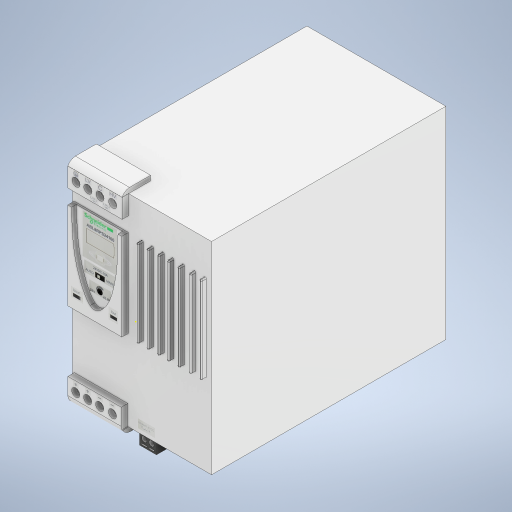
# Autodesk Inventor part: napojna_jedinica_ABL8RPS24100
Saved by Autodesk Inventor 2023 (Build 270158000, 158)
## iProperties
Created: 2022-07-15
Part Number: napojna_jedinica_ABL8RPS24100
Material: Generic
Document SubType Name: Sheet Metal
Designer: User
Density: 1 g/cm^3
Sheet Metal Rule: Default
Appearance: Default
Author: User
Autodesk Inventor part; units mm, degrees
ref_plane "YZ Plane" through (0, 0, 0) normal (1, 0, 0) x (0, 1, 0)
ref_plane "XZ Plane" through (0, 0, 0) normal (0, 1, 0) x (-1, 0, 0)
ref_plane "XY Plane" through (0, 0, 0) normal (0, 0, 1) x (1, 0, 0)
sketch "Sketch1" plane through (0, 0, 0) normal (0, 0, 1) x (1, 0, 0)
  line L0 (43, -62.5) -> (-43, -62.5)
  line L1 (-43, -62.5) -> (-43, 62.5)
  line L2 (-43, 62.5) -> (43, 62.5)
  line L3 (43, 62.5) -> (43, -62.5)
  line L4 (43, -62.5) -> (-43, 62.5) construction
  line L5 (-43, -62.5) -> (43, 62.5) construction
  point P0 (0, 0)
  dimension "d0" = 125
  dimension "d1" = 86
  constraints: 12 end point, 2 midpoint, 2 parallel, 1 horizontal, 1 perpendicular
  measures "d0" distance of L0.end L1.end
  measures "d1" distance of L1.end L2.end
extrude "Extrusion1" add sketch "Sketch1" against normal blind 145
sketch "Sketch2" plane through (0, 0, 0) normal (0, 0, 1) x (1, 0, 0)
  line L0 (-8.4534, -12.4164) -> (-42.0011, -12.4164)
  line L1 (-42.0011, -12.4164) -> (-42.0011, 41.6134)
  line L2 (-42.0011, 41.6134) -> (-8.4534, 41.6134)
  line L3 (-8.4534, 41.6134) -> (-8.4534, -12.4164)
  line L4 (-8.4534, -12.4164) -> (-42.0011, 41.6134) construction
  line L5 (-42.0011, -12.4164) -> (-8.4534, 41.6134) construction
  line L6 (-8.3237, 50.7106) -> (-41.8747, 50.7106)
  line L7 (-41.8747, 50.7106) -> (-41.8747, 62.4919)
  line L8 (-41.8747, 62.4919) -> (-8.3237, 62.4919)
  line L9 (-8.3237, 62.4919) -> (-8.3237, 50.7106)
  line L10 (-8.3237, 50.7106) -> (-41.8747, 62.4919) construction
  line L11 (-41.8747, 50.7106) -> (-8.3237, 62.4919) construction
  line L12 (-41.8747, -50.1984) -> (-8.8359, -50.1984)
  line L13 (-8.8359, -50.1984) -> (-8.8359, -62.748)
  line L14 (-8.8359, -62.748) -> (-41.8747, -62.748)
  line L15 (-41.8747, -62.748) -> (-41.8747, -50.1984)
  line L16 (-41.8747, -50.1984) -> (-8.8359, -62.748) construction
  line L17 (-8.8359, -50.1984) -> (-41.8747, -62.748) construction
  line L18 (0.7683, -12.3428) -> (-0.7683, -12.3428)
  line L19 (-0.7683, -12.3428) -> (-0.7683, 41.6871)
  line L20 (-0.7683, 41.6871) -> (0.7683, 41.6871)
  line L21 (0.7683, 41.6871) -> (0.7683, -12.3428)
  line L22 (0.7683, -12.3428) -> (-0.7683, 41.6871) construction
  line L23 (-0.7683, -12.3428) -> (0.7683, 41.6871) construction
  line L24 (26.2391, -12.3428) -> (24.7024, -12.3428)
  line L25 (24.7024, -12.3428) -> (24.7024, 41.6871)
  line L26 (24.7024, 41.6871) -> (26.2391, 41.6871)
  line L27 (26.2391, 41.6871) -> (26.2391, -12.3428)
  line L28 (26.2391, -12.3428) -> (24.7024, 41.6871) construction
  line L29 (24.7024, -12.3428) -> (26.2391, 41.6871) construction
  line L30 (19.7125, -12.3729) -> (18.1758, -12.3729)
  line L31 (18.1758, -12.3729) -> (18.1758, 41.7648)
  line L32 (18.1758, 41.7648) -> (19.7125, 41.7648)
  line L33 (19.7125, 41.7648) -> (19.7125, -12.3729)
  line L34 (19.7125, -12.3729) -> (18.1758, 41.7648) construction
  line L35 (18.1758, -12.3729) -> (19.7125, 41.7648) construction
  line L36 (33.3265, -12.2364) -> (31.7898, -12.2364)
  line L37 (31.7898, -12.2364) -> (31.7898, 41.6856)
  line L38 (31.7898, 41.6856) -> (33.3265, 41.6856)
  line L39 (33.3265, 41.6856) -> (33.3265, -12.2364)
  line L40 (33.3265, -12.2364) -> (31.7898, 41.6856) construction
  line L41 (31.7898, -12.2364) -> (33.3265, 41.6856) construction
  line L42 (5.5817, 41.7558) -> (7.1183, 41.7558)
  line L43 (5.5817, -12.3819) -> (5.5817, 41.7558)
  line L44 (7.1183, 41.7558) -> (7.1183, -12.3819)
  line L45 (5.5817, -12.3819) -> (7.1183, 41.7558) construction
  line L46 (7.1183, -12.3819) -> (5.5817, 41.7558) construction
  line L47 (7.1183, -12.3819) -> (5.5817, -12.3819)
  line L48 (38.2302, 41.6103) -> (39.7669, 41.6103)
  line L49 (38.2302, -12.3118) -> (38.2302, 41.6103)
  line L50 (39.7669, 41.6103) -> (39.7669, -12.3118)
  line L51 (38.2302, -12.3118) -> (39.7669, 41.6103) construction
  line L52 (39.7669, -12.3118) -> (38.2302, 41.6103) construction
  line L53 (39.7669, -12.3118) -> (38.2302, -12.3118)
  line L54 (12.1537, 41.8636) -> (13.6904, 41.8636)
  line L55 (12.1537, -12.2741) -> (12.1537, 41.8636)
  line L56 (13.6904, 41.8636) -> (13.6904, -12.2741)
  line L57 (12.1537, -12.2741) -> (13.6904, 41.8636) construction
  line L58 (13.6904, -12.2741) -> (12.1537, 41.8636) construction
  line L59 (13.6904, -12.2741) -> (12.1537, -12.2741)
  point P0 (0, 0)
  point P1 (-25.2272, 14.5985)
  point P2 (-25.0992, 56.6012)
  point P3 (-25.3553, -56.4732)
  point P4 (0, 14.6721)
  point P5 (1.5875, 1.5875)
  point P6 (25.4708, 14.6721)
  point P7 (3.175, 3.175)
  point P8 (18.9442, 14.696)
  point P9 (4.7625, 4.7625)
  point P10 (32.5581, 14.7246)
  point P11 (3.175, 3.175)
  point P12 (6.35, 14.6869)
  point P13 (4.7625, 4.7625)
  point P14 (38.9985, 14.6493)
  point P15 (6.35, 6.35)
  point P16 (12.9221, 14.7948)
  constraints: 120 end point, 20 midpoint, 20 parallel, 10 horizontal, 10 perpendicular
extrude "Extrusion2" add sketch "Sketch2" along normal blind 4 contours L0 L1 L2 L3
extrude "Extrusion3" add sketch "Sketch2" along normal blind 4 contours L6 L7 L8 L9 | L12 L13 L14 L15
extrude "Extrusion4" add sketch "Sketch2" along normal blind 3 contours L18 L19 L20 L21 | L24 L25 L26 L27 | L30 L31 L32 L33 | L36 L37 L38 L39 | L42 L44 L47 L43 | L48 L50 L53 L49 | L54 L56 L59 L55
fillet "Fillet1" radius 0.7 2 edges at (0.7683, 14.6721, 3) (-0.7683, 14.6721, 3)
fillet "Fillet2" radius 0.7 12 edges at (5.5817, 14.6869, 3) (7.1183, 14.6869, 3) (12.1537, 14.7948, 3) (13.6904, 14.7948, 3) (18.1758, 14.696, 3) (19.7125, 14.696, 3) (24.7024, 14.6721, 3) (26.2391, 14.6721, 3) (31.7898, 14.7246, 3) (33.3265, 14.7246, 3) (38.2302, 14.6493, 3) (39.7669, 14.6493, 3)
fillet "Fillet3" radius 0.7 35 edges at (38.9985, 41.6103, 3) (38.4352, 41.6103, 2.795) (38.2302, 41.6103, 1.15) (39.7669, 41.6103, 1.15) (39.5618, 41.6103, 2.795) (32.5581, 41.6856, 3) (31.9948, 41.6856, 2.795) (31.7898, 41.6856, 1.15) (33.3265, 41.6856, 1.15) (33.1215, 41.6856, 2.795) (25.4708, 41.6871, 3) (24.9075, 41.6871, 2.795) (24.7024, 41.6871, 1.15) (26.2391, 41.6871, 1.15) (26.0341, 41.6871, 2.795) (18.9442, 41.7648, 3) (18.3809, 41.7648, 2.795) (18.1758, 41.7648, 1.15) (19.7125, 41.7648, 1.15) (19.5075, 41.7648, 2.795) (12.9221, 41.8636, 3) (12.3588, 41.8636, 2.795) (12.1537, 41.8636, 1.15) (13.6904, 41.8636, 1.15) (13.4854, 41.8636, 2.795) (6.35, 41.7558, 3) (5.7867, 41.7558, 2.795) (5.5817, 41.7558, 1.15) (7.1183, 41.7558, 1.15) (6.9133, 41.7558, 2.795) (0, 41.6871, 3) (-0.5633, 41.6871, 2.795) (-0.7683, 41.6871, 1.15) (0.7683, 41.6871, 1.15) (0.5633, 41.6871, 2.795)
fillet "Fillet4" radius 0.7 35 edges at (0.7683, -12.3428, 1.15) (0, -12.3428, 3) (-0.5633, -12.3428, 2.795) (-0.7683, -12.3428, 1.15) (0.5633, -12.3428, 2.795) (7.1183, -12.3819, 1.15) (6.35, -12.3819, 3) (5.7867, -12.3819, 2.795) (5.5817, -12.3819, 1.15) (6.9133, -12.3819, 2.795) (13.6904, -12.2741, 1.15) (12.9221, -12.2741, 3) (12.3588, -12.2741, 2.795) (12.1537, -12.2741, 1.15) (13.4854, -12.2741, 2.795) (19.7125, -12.3729, 1.15) (18.9442, -12.3729, 3) (18.3809, -12.3729, 2.795) (18.1758, -12.3729, 1.15) (19.5075, -12.3729, 2.795) (24.9075, -12.3428, 2.795) (25.4708, -12.3428, 3) (26.0341, -12.3428, 2.795) (26.2391, -12.3428, 1.15) (24.7024, -12.3428, 1.15) (33.3265, -12.2364, 1.15) (32.5581, -12.2364, 3) (31.9948, -12.2364, 2.795) (31.7898, -12.2364, 1.15) (33.1215, -12.2364, 2.795) (39.7669, -12.3118, 1.15) (38.9985, -12.3118, 3) (38.4352, -12.3118, 2.795) (38.2302, -12.3118, 1.15) (39.5618, -12.3118, 2.795)
sketch "Sketch3" plane through (-43, 62.5, 0) normal (0, 1, 0) x (1, 0, 0)
  line L0 (34.6244, -3.9581) -> (1.0619, -3.9581)
  line L1 (1.0619, -3.9581) -> (1.0619, 13.6548)
  line L2 (1.0619, 13.6548) -> (34.6244, 13.6548)
  line L3 (34.6244, 13.6548) -> (34.6244, -3.9581)
  line L4 (34.6244, -3.9581) -> (1.0619, 13.6548) construction
  line L5 (1.0619, -3.9581) -> (34.6244, 13.6548) construction
  point P0 (43, 0)
  point P1 (17.8432, 4.8484)
  constraints: 12 end point, 2 midpoint, 2 parallel, 1 horizontal, 1 perpendicular
extrude "Extrusion5" add sketch "Sketch3" along normal blind 3
fillet "Fillet5" radius 5 1 edges at (-25.1568, 65.5, 3.9581)
sketch "Sketch4" plane through (-43, -62.5, -145) normal (0, -1, 0) x (1, 0, 0)
  line L0 (34.5466, 149) -> (0.9989, 149) projected
  line L1 (34.6874, 128.9171) -> (0.9989, 128.9171)
  line L2 (0.9989, 128.9171) -> (0.9989, 149)
  line L3 (0.9989, 149) -> (34.6874, 149)
  line L4 (34.6874, 149) -> (34.6874, 128.9171)
  line L5 (34.6874, 128.9171) -> (0.9989, 149) construction
  line L6 (0.9989, 128.9171) -> (34.6874, 149) construction
  point P0 (43, 145)
  point P1 (17.8432, 138.9585)
  constraints: 12 end point, 2 midpoint, 2 parallel, 1 horizontal, 1 perpendicular
extrude "Extrusion6" add sketch "Sketch4" along normal blind 3
fillet "Fillet6" radius 5 1 edges at (-25.1568, -65.5, 4)
sketch "Sketch5" plane through (0, 0, 4) normal (0, 0, 1) x (1, 0, 0)
  point P0 (0, 0)
sketch "Sketch6" plane through (0, 0, 4) normal (0, 0, 1) x (1, 0, 0)
  line L0 (-42.0134, 40.8092) -> (-7.5398, 40.8092) construction
  line L1 (-7.5398, 40.8092) -> (-7.5398, -8.8157) construction
  line L2 (-7.5398, -8.8157) -> (-42.0134, -8.8157) construction
  line L3 (-42.0134, -8.8157) -> (-42.0134, 40.8092) construction
  line L4 (-42.0011, 41.6134) -> (-8.4534, 41.6134) projected
  spline S0 degree 4 poles (-39.6427, 41.6134) (-39.5386, 39.0441) (-39.1974, 21.8727) (-37.9398, 12.4752) (-31.2758, -3.0074) (-28.1197, -5.3577) knots 0 0 0 0 0 0.490778 1 1 1 1 1
  spline S1 degree 4 poles (-10.883, 41.6134) (-10.9429, 39.1847) (-10.7419, 26.6675) (-12.0599, 17.1608) (-16.3516, -0.707) (-22.8529, -6.5254) (-25.813, -7.2256) (-28.1197, -5.3577) knots 0 0 0 0 0 0.398035 0.568703 0.718295 1 1 1 1 1
  line L5 (-39.6427, 41.6134) -> (-10.883, 41.6134)
  point P0 (0, 0)
  point P1 (-39.4451, 35.6169)
  point P2 (-38.6549, 23.4672)
  point P3 (-36.5806, 12.1076)
  point P4 (-32.4319, 0.8469)
  point P5 (-10.9341, 35.6169)
  point P6 (-11.5549, 23.4671)
  point P7 (-13.4008, 12.1076)
  point P8 (-17.2522, 0.8469)
  point P9 (-22.0273, -4.981)
  point P10 (-25.2273, -6.4217)
  constraints: 2 end point, 2 point on line, 1 collinear, 16 other
extrude "Extrusion7" cut sketch "Sketch6" against normal blind 3
sketch "Sketch7" plane through (0, 0, 1) normal (0, 0, 1) x (1, 0, 0)
  line L0 (-35.8459, 40.4822) -> (-14.5747, 40.4822) construction
  line L1 (-14.5747, 40.4822) -> (-14.5747, 15.9143) construction
  line L2 (-14.5747, 15.9143) -> (-35.8459, 15.9143) construction
  line L3 (-35.8459, 15.9143) -> (-35.8459, 40.4822) construction
  line L4 (-34.7955, 14.6387) -> (-15.0999, 14.6387) construction
  line L5 (-15.0999, 14.6387) -> (-15.0999, 7.9537) construction
  line L6 (-15.0999, 7.9537) -> (-34.7955, 7.9537) construction
  line L7 (-34.7955, 7.9537) -> (-34.7955, 14.6387) construction
  line L8 (-31.6442, 5.4452) -> (-18.2512, 5.4452) construction
  line L9 (-18.2512, 5.4452) -> (-18.2512, -0.4276) construction
  line L10 (-18.2512, -0.4276) -> (-31.6442, -0.4276) construction
  line L11 (-31.6442, -0.4276) -> (-31.6442, 5.4452) construction
  point P0 (0, 0)
  constraints: 6 other
decal "Decal1"
decal "Decal2"
decal "Decal3"
sketch "Sketch8" plane through (0, 0, 4) normal (0, 0, 1) x (1, 0, 0)
  line L0 (-16.7418, -0.0611) -> (-10.8655, -0.0611) construction
  line L1 (-10.8655, -0.0611) -> (-10.8655, -6.9406) construction
  line L2 (-10.8655, -6.9406) -> (-16.7418, -6.9406) construction
  line L3 (-16.7418, -6.9406) -> (-16.7418, -0.0611) construction
  line L4 (-39.8987, -0.6259) -> (-32.597, -0.6259) construction
  line L5 (-32.597, -0.6259) -> (-32.597, -6.5585) construction
  line L6 (-32.597, -6.5585) -> (-39.8987, -6.5585) construction
  line L7 (-39.8987, -6.5585) -> (-39.8987, -0.6259) construction
  point P0 (0, 0)
  constraints: 4 other
decal "Decal4"
decal "Decal5"
sketch "Sketch9" plane through (0, 0, 4) normal (0, 0, 1) x (1, 0, 0)
  circle A0 centre (-36.8873, 56.3383) radius 2.54
  circle A1 centre (-29.4981, 56.3383) radius 2.54
  circle A2 centre (-22.0468, 56.3383) radius 2.54
  circle A3 centre (-14.1608, 56.3383) radius 2.54
  point P0 (0, 0)
  dimension "d117" = 5.08
  dimension "d118" = 5.08
  dimension "d119" = 5.08
  dimension "d120" = 5.08
  constraints: 4 centre point
  measures "d117" diameter of A0
  measures "d118" diameter of A1
  measures "d119" diameter of A2
  measures "d120" diameter of A3
sketch "Sketch10" plane through (0, 0, 4) normal (0, 0, 1) x (1, 0, 0)
  circle A0 centre (-37.0437, -56.4262) radius 2.54
  circle A1 centre (-29.6545, -56.4262) radius 2.54
  circle A2 centre (-22.2032, -56.4262) radius 2.54
  circle A3 centre (-14.3172, -56.4262) radius 2.54
  point P0 (0, 0)
  dimension "d121" = 5.08
  dimension "d122" = 5.08
  dimension "d123" = 5.08
  dimension "d124" = 5.08
  constraints: 4 centre point
  measures "d121" diameter of A0
  measures "d122" diameter of A1
  measures "d123" diameter of A2
  measures "d124" diameter of A3
extrude "Extrusion8" cut sketch "Sketch9" against normal blind 3
extrude "Extrusion9" cut sketch "Sketch10" against normal blind 3
sketch "Sketch11" plane through (0, 0, 4) normal (0, 0, 1) x (1, 0, 0)
  line L0 (-31.3238, -50.4843) -> (-27.885, -50.4843) construction
  line L1 (-27.885, -50.4843) -> (-27.885, -53.5793) construction
  line L2 (-27.885, -53.5793) -> (-31.3238, -53.5793) construction
  line L3 (-31.3238, -53.5793) -> (-31.3238, -50.4843) construction
  line L4 (-38.6549, -50.5658) -> (-35.3066, -50.5658) construction
  line L5 (-35.3066, -50.5658) -> (-35.3066, -53.5793) construction
  line L6 (-35.3066, -53.5793) -> (-38.6549, -53.5793) construction
  line L7 (-38.6549, -53.5793) -> (-38.6549, -50.5658) construction
  line L8 (-16.3901, -50.587) -> (-12.4983, -50.587) construction
  line L9 (-12.4983, -50.587) -> (-12.4983, -53.2729) construction
  line L10 (-12.4983, -53.2729) -> (-16.3901, -53.2729) construction
  line L11 (-16.3901, -53.2729) -> (-16.3901, -50.587) construction
  line L12 (-24.1737, -50.656) -> (-20.1914, -50.656) construction
  line L13 (-20.1914, -50.656) -> (-20.1914, -53.4044) construction
  line L14 (-20.1914, -53.4044) -> (-24.1737, -53.4044) construction
  line L15 (-24.1737, -53.4044) -> (-24.1737, -50.656) construction
  point P0 (0, 0)
  constraints: 8 other
decal "Decal6"
decal "Decal7"
decal "Decal8"
decal "Decal9"
sketch "Sketch12" plane through (0, 0, 4) normal (0, 0, 1) x (1, 0, 0)
  line L0 (-28.2409, 53.9392) -> (-23.087, 53.9392) construction
  line L1 (-23.087, 53.9392) -> (-23.087, 50.9022) construction
  line L2 (-23.087, 50.9022) -> (-28.2409, 50.9022) construction
  line L3 (-28.2409, 50.9022) -> (-28.2409, 53.9392) construction
  line L4 (-20.5627, 54.083) -> (-15.6193, 54.083) construction
  line L5 (-15.6193, 54.083) -> (-15.6193, 50.999) construction
  line L6 (-15.6193, 50.999) -> (-20.5627, 50.999) construction
  line L7 (-20.5627, 50.999) -> (-20.5627, 54.083) construction
  line L8 (-38.7589, 62.1024) -> (-34.9724, 62.1024) construction
  line L9 (-34.9724, 62.1024) -> (-34.9724, 58.9802) construction
  line L10 (-34.9724, 58.9802) -> (-38.7589, 58.9802) construction
  line L11 (-38.7589, 58.9802) -> (-38.7589, 62.1024) construction
  line L12 (-31.5015, 62.0586) -> (-27.3994, 62.0586) construction
  line L13 (-27.3994, 62.0586) -> (-27.3994, 59.1872) construction
  line L14 (-27.3994, 59.1872) -> (-31.5015, 59.1872) construction
  line L15 (-31.5015, 59.1872) -> (-31.5015, 62.0586) construction
  line L16 (-23.6129, 62.215) -> (-20.0368, 62.215) construction
  line L17 (-20.0368, 62.215) -> (-20.0368, 59.0954) construction
  line L18 (-20.0368, 59.0954) -> (-23.6129, 59.0954) construction
  line L19 (-23.6129, 59.0954) -> (-23.6129, 62.215) construction
  line L20 (-16.4607, 62.2829) -> (-11.5172, 62.2829) construction
  line L21 (-11.5172, 62.2829) -> (-11.5172, 59.2924) construction
  line L22 (-11.5172, 59.2924) -> (-16.4607, 59.2924) construction
  line L23 (-16.4607, 59.2924) -> (-16.4607, 62.2829) construction
  point P0 (0, 0)
  constraints: 12 other
decal "Decal10"
decal "Decal11"
decal "Decal12"
decal "Decal13"
decal "Decal14"
decal "Decal15"
sketch "Sketch13" plane through (-43, -62.5, -145) normal (0, -1, 0) x (1, 0, 0)
  line L0 (40.7571, 144.3568) -> (51.2581, 144.3568)
  line L1 (51.2581, 144.3568) -> (51.2581, 130.5653)
  line L2 (51.2581, 130.5653) -> (40.7571, 130.5653)
  line L3 (40.7571, 130.5653) -> (40.7571, 144.3568)
  line L4 (40.7571, 144.3568) -> (51.2581, 130.5653) construction
  line L5 (51.2581, 144.3568) -> (40.7571, 130.5653) construction
  point P0 (43, 145)
  point P1 (46.0076, 137.4611)
  constraints: 12 end point, 2 midpoint, 2 parallel, 1 horizontal, 1 perpendicular
extrude "Extrusion10" add sketch "Sketch13" along normal blind 7
sketch "Sketch14" plane through (-2.2429, -62.5, -0.6432) normal (0, 0, 1) x (1, 0, 0)
  circle A0 centre (2.9605, -2.391) radius 1.6234
  circle A1 centre (7.5433, -2.391) radius 1.6234
  line L0 (4.5839, -6.021) -> (1.3371, -6.021)
  line L1 (1.3371, -6.021) -> (1.3371, -5.295)
  line L2 (1.3371, -5.295) -> (4.5839, -5.295)
  line L3 (4.5839, -5.295) -> (4.5839, -6.021)
  line L4 (4.5839, -6.021) -> (1.3371, -5.295) construction
  line L5 (1.3371, -6.021) -> (4.5839, -5.295) construction
  line L6 (9.1667, -6.021) -> (5.9199, -6.021)
  line L7 (5.9199, -6.021) -> (5.9199, -5.295)
  line L8 (5.9199, -5.295) -> (9.1667, -5.295)
  line L9 (9.1667, -5.295) -> (9.1667, -6.021)
  line L10 (9.1667, -6.021) -> (5.9199, -5.295) construction
  line L11 (5.9199, -6.021) -> (9.1667, -5.295) construction
  point P0 (2.2429, 62.5)
  point P1 (2.9605, -5.658)
  point P2 (7.5433, -5.658)
  constraints: 24 end point, 4 midpoint, 4 parallel, 2 centre point, 2 horizontal, 2 perpendicular
extrude "Extrusion11" cut sketch "Sketch14" against normal blind 7 contours A0 | A1
extrude "Extrusion12" cut sketch "Sketch14" against normal blind 4 contours L0 L1 L2 L3 | L6 L7 L8 L9
sketch "Sketch15" plane through (0, 0, 0) normal (0, 0, 1) x (1, 0, 0)
  line L0 (-2.6171, -55.0352) -> (8.0827, -55.0352) construction
  line L1 (8.0827, -55.0352) -> (8.0827, -60.2592) construction
  line L2 (8.0827, -60.2592) -> (-2.6171, -60.2592) construction
  line L3 (-2.6171, -60.2592) -> (-2.6171, -55.0352) construction
  point P0 (0, 0)
  constraints: 2 other
decal "Decal16"
body "Solid1"
